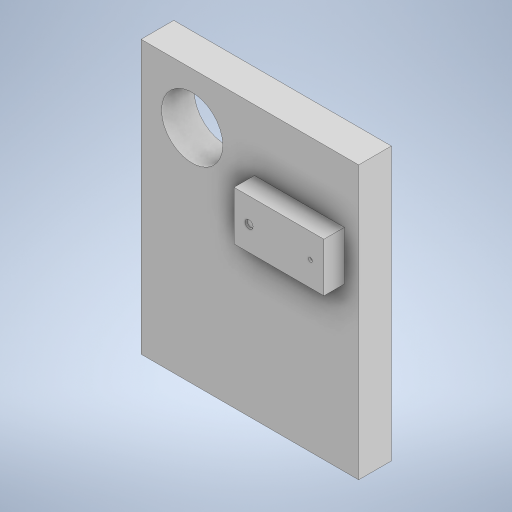
# Autodesk Inventor part: senzor
Saved by Autodesk Inventor 2023 (Build 270158000, 158)
## iProperties
Created: 2023-05-23
Part Number: senzor
Material: Všeobecné
Document SubType Name: Modeling
Designer: Simak
Density: 1 g/cm^3
Appearance: Výchozí
Author: Simak
Autodesk Inventor part; units mm, degrees
ref_plane "YZ Plane" through (0, 0, 0) normal (1, 0, 0) x (0, 1, 0)
ref_plane "XZ Plane" through (0, 0, 0) normal (0, 1, 0) x (-1, 0, 0)
ref_plane "XY Plane" through (0, 0, 0) normal (0, 0, 1) x (1, 0, 0)
sketch "Náčrt1" plane through (0, 0, 0) normal (0, 0, 1) x (1, 0, 0)
  line L0 (-10.65, 0) -> (0, 0)
  line L1 (0, 0) -> (0, -13.35)
  line L2 (0, -13.35) -> (-10.65, -13.35)
  line L3 (-10.65, -13.35) -> (-10.65, 0)
  circle A0 centre (-8.15, -2.5) radius 1.5
  dimension "d0" = 10.65
  dimension "d1" = 13.35
  dimension "d2" = 3
  dimension "d3" = 1
  dimension "d4" = 1
  constraints: 8 end point, 2 parallel, 1 centre point, 1 coincident, 1 horizontal, 1 perpendicular
  measures "d0" distance of L0.start L0.end
  measures "d1" distance of L0.end L1.end
  measures "d2" diameter of A0
  measures "d3" distance edge to line of A0 L0
  measures "d4" distance edge to line of A0 L3
extrude "Vysunutí1" add sketch "Náčrt1" along normal blind 1.6
sketch "Náčrt2" plane through (0, 0, 1.6) normal (0, 0, 1) x (1, 0, 0)
  line L0 (-5.1, -3) -> (-0.7, -3)
  line L1 (-0.7, -3) -> (-0.7, -5.4)
  line L2 (-0.7, -5.4) -> (-5.1, -5.4)
  line L3 (-5.1, -5.4) -> (-5.1, -3)
  point P0 (0, 0)
  dimension "d7" = 2.4
  dimension "d8" = 4.4
  dimension "d9" = 3
  dimension "d10" = 0.7
  constraints: 8 end point, 2 parallel, 1 horizontal, 1 perpendicular
  measures "d7" distance of L0.end L1.end
  measures "d8" distance of L0.start L0.end
  measures "d9" distance from line of L0 point (0, 0)
  measures "d10" distance from line of point (0, 0) L1
extrude "Vysunutí2" add sketch "Náčrt2" along normal blind 1
sketch "Náčrt3" plane through (0, 0, 2.6) normal (0, 0, 1) x (1, 0, 0)
  circle A0 centre (-4.365, -4.2) radius 0.2
  circle A1 centre (-1.365, -4.2) radius 0.1
  line L0 (-5.1, -3) -> (-5.1, -5.4) projected
  line L1 (-0.7, -5.4) -> (-0.7, -3) projected
  point P0 (0, 0)
  point P1 (-5.1, -4.2)
  point P2 (-0.7, -4.2)
  dimension "d13" = 0.4
  dimension "d14" = 0.2
  dimension "d16" = 0.665
  dimension "d17" = 3
  constraints: 2 centre point, 2 horizontal alignment, 2 midpoint
  measures "d13" diameter of A0
  measures "d14" diameter of A1
  measures "d16" distance from line of L1 A1.centre
  measures "d17" distance of A1.centre A0.centre
extrude "Vysunutí3" cut sketch "Náčrt3" against normal blind 0.1
